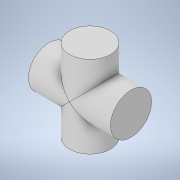
# Autodesk Inventor part: U_Joint_Center
Saved by Autodesk Inventor 2020.1 (Build 241239000, 239)
## iProperties
Created: 2019-10-27
Part Number: U_Joint_Center
Material: Generic
Document SubType Name: Modeling
Designer: sshel
Density: 1 g/cm^3
Appearance: Default
Mass: 2474.93 g
Surface Area: 1170.8 cm^2
Volume: 2474.93 cm^3
Author: sshel
Autodesk Inventor part; units mm, degrees
ref_plane "YZ Plane" through (0, 0, 0) normal (1, 0, 0) x (0, 1, 0)
ref_plane "XZ Plane" through (0, 0, 0) normal (0, 1, 0) x (-1, 0, 0)
ref_plane "XY Plane" through (0, 0, 0) normal (0, 0, 1) x (1, 0, 0)
sketch "Sketch1" plane through (0, 0, 0) normal (0, 0, 1) x (1, 0, 0)
  circle A0 centre (0, 0) radius 200
  dimension "d7" = 200
  constraints: 1 centre point, 1 coincident
  measures "d7" radius of A0
extrude "Extrusion1" add sketch "Sketch1" along normal mid plane 800
sketch "Sketch2" plane through (0, 0, 0) normal (0, 1, 0) x (-1, 0, 0)
  circle A0 centre (0, 0) radius 200
  dimension "d8" = 200
  constraints: 1 centre point, 1 coincident
  measures "d8" radius of A0
extrude "Extrusion2" add sketch "Sketch2" along normal mid plane 800
equation "\"d7\" = rod_radius"
equation "\"d1\" = U_length"
equation "\"d8\" = rod_radius"
equation "\"d4\" = U_length"
equation "\"rod_radius\" = 200"
equation "\"U_length\" = 4 * rod_radius"
body "Solid1"
